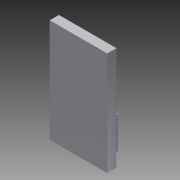
# Autodesk Inventor part: RumbaBoard
Saved by Autodesk Inventor 2015 SP1 (Build 190203100, 203)
## iProperties
Created: 2014-10-19
Part Number: RumbaBoard
Material: Generic
Document SubType Name: Modeling
Designer: Jack
Density: 1 g/cm^3
Appearance: Smooth - White
Mass: 122.256 g
Surface Area: 268.38 cm^2
Volume: 122.256 cm^3
Author: Jack
Autodesk Inventor part; units mm, degrees
ref_plane "YZ Plane" through (0, 0, 0) normal (1, 0, 0) x (0, 1, 0)
ref_plane "XZ Plane" through (0, 0, 0) normal (0, 1, 0) x (-1, 0, 0)
ref_plane "XY Plane" through (0, 0, 0) normal (0, 0, 1) x (1, 0, 0)
sketch "Sketch1" plane through (0, 0, 0) normal (0, 1, 0) x (-1, 0, 0)
  line L0 (0, 0) -> (75, 0)
  line L1 (75, 0) -> (75, -135)
  line L2 (75, -135) -> (0, -135)
  line L3 (0, -135) -> (0, 0)
  dimension "d0" = 75
  dimension "d1" = 135
  constraints: 8 end point, 2 parallel, 1 horizontal, 1 perpendicular
  measures "d0" distance of L1.end L2.end
  measures "d1" distance of L0.end L1.end
extrude "Extrusion1" add sketch "Sketch1" along normal blind 12
sketch "Sketch4" plane through (0, 12, 0) normal (0, 1, 0) x (1, 0, 0)
  line L0 (0, 0) -> (0, 135) projected
  line L1 (0, 135) -> (-75, 135) projected
  line L2 (-16, 133) -> (-17, 133)
  line L3 (-17, 133) -> (-17, 91)
  line L4 (-17, 91) -> (-16, 91)
  line L5 (-16, 91) -> (-16, 133)
  dimension "d10" = 1
  dimension "d11" = 42
  dimension "d12" = 16
  dimension "d13" = 2
  constraints: 8 end point, 2 parallel, 1 horizontal, 1 perpendicular
  measures "d10" distance of L4.end L3.end
  measures "d11" distance of L3.end L2.end
  measures "d12" distance between parallel lines of L0 L5
  measures "d13" distance between parallel lines of L1 L2
extrude "Extrusion3" add sketch "Sketch4" along normal blind 18
body "Solid1"
